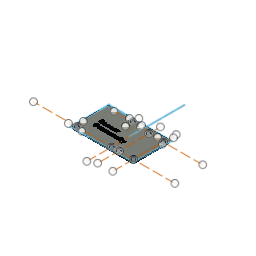
Luftdaten_sensor_holder (Autodesk Fusion 360 design; units mm, degrees)
Autodesk Fusion 360 part; units mm, degrees
sketch "Sketch1" plane through (0, 0, 0) normal (0, 1, 0) x (1, 0, 0)
  circle A0 centre (32.103, -20.4759) radius 1.325
  circle A1 centre (92.103, -20.4759) radius 1.325
  circle A2 centre (73.103, 34.5241) radius 1.325
  line L0 (100.7373, -20.4759) -> (-42.1485, -20.4759) construction
  circle A3 centre (73.103, 34.5241) radius 2.325
  circle A4 centre (92.103, -20.4759) radius 2.325
  circle A5 centre (32.103, -20.4759) radius 2.325
  circle A6 centre (104.103, 31.0241) radius 1.325
  circle A7 centre (129.103, 31.0241) radius 1.325
  circle A8 centre (104.103, -20.4759) radius 1.325
  circle A9 centre (129.103, -20.4759) radius 1.325
  line L1 (104.103, 50.9293) -> (104.103, -56.6428) construction
  line L2 (129.103, -55.7039) -> (129.103, 53.0753) construction
  circle A10 centre (104.103, 31.0241) radius 2.325
  circle A11 centre (104.103, -20.4759) radius 2.325
  circle A12 centre (129.103, -20.4759) radius 2.325
  circle A13 centre (129.103, 31.0241) radius 2.325
  line L3 (196.6906, 31.0241) -> (105, 31.0241) construction
  line L4 (200.3141, -20.4759) -> (105.3141, -20.4759) construction
  line L5 (92.103, -63.1974) -> (92.103, 103.9329) construction
  line L6 (92.103, 103.9329) -> (92.103, 10)
  line L7 (71.8078, 34.4241) -> (41, 34.4241) construction
  line L8 (73.103, 22) -> (73.103, 45) construction
  line L9 (134.428, -25.8009) -> (26.778, -25.8009)
  line L10 (26.778, -25.8009) -> (26.778, 39.8491)
  line L11 (26.778, 39.8491) -> (134.428, 39.8491)
  line L12 (134.428, 39.8491) -> (134.428, -25.8009)
  line L13 (29.778, -7) -> (29.778, -20.4759) construction
  line L14 (20, -22.8009) -> (43, -22.8009) construction
  line L15 (87, 33.3491) -> (117, 33.3491) construction
  line L16 (131.428, 46) -> (131.428, 27) construction
  line L17 (86, 36.8491) -> (65, 36.8491) construction
  dimension "d1" = 2.65
  dimension "d3" = 2.65
  dimension "d4" = 2.65
  dimension "d5" = 60
  dimension "d10" = 41
  dimension "d11" = 55
  dimension "d13" = 1
  dimension "d14" = 1
  dimension "d15" = 1
  dimension "d18" = 2.65
  dimension "d19" = 2.65
  dimension "d20" = 2.65
  dimension "d21" = 2.65
  dimension "d22" = 1
  dimension "d23" = 1
  dimension "d24" = 1
  dimension "d25" = 1
  dimension "d26" = 25
  dimension "d27" = 51.5
  dimension "d28" = 12
  dimension "d31" = 3
  dimension "d32" = 3
  dimension "d34" = 3
  dimension "d42" = 3
  constraint horizontal L0
  constraint coincident A0.centre L0
  constraint coincident A1.centre L0
  constraint vertical L1
  constraint vertical L2
  constraint coincident A7.centre L2
  constraint coincident A9.centre L2
  constraint coincident A8.centre L1
  constraint coincident A6.centre L1
  constraint horizontal L3
  constraint coincident A6.centre L3
  constraint coincident A7.centre L3
  constraint horizontal L4
  constraint coincident A8.centre L4
  constraint coincident A9.centre L4
  constraint perpendicular L0 L5
  constraint coincident L5 L6.end
  constraint coincident A1.centre L5
  constraint horizontal L7
  constraint vertical L8
  constraint coincident A2.centre L8
  constraint horizontal L9
  constraint vertical L10
  constraint horizontal L11
  constraint vertical L12
  constraint coincident L0 L13.end
  constraint perpendicular L0 L13
  constraint tangent A5 L13
  constraint perpendicular L10 L14
  constraint tangent A5 L14
  constraint perpendicular L5 L15
  constraint tangent A10 L15
  constraint perpendicular L11 L16
  constraint tangent A13 L16
  constraint collinear L0 L4
  constraint horizontal L17
  constraint tangent A3 L17
  measures "d1" diameter of A2
  measures "d3" diameter of A0
  measures "d4" diameter of A1
  measures "d5" distance of A0.centre A1.centre
  measures "d10" horizontal distance of A0.centre A2.centre
  measures "d11" vertical distance of A0.centre A2.centre
  measures "d18" diameter of A6
  measures "d19" diameter of A7
  measures "d20" diameter of A8
  measures "d21" diameter of A9
  measures "d26" distance of L1 L2
  measures "d27" distance of L3 L4
  measures "d28" horizontal distance of A1.centre A6.centre
  measures "d31" distance of L10 L13
  measures "d32" distance of L9 L14
  measures "d34" distance of L12 L16
  measures "d42" distance of L11 L17
extrude "Extrude2" add sketch "Sketch1" against normal blind 1.5 contours A0 | A1 | A2 | A3 | A4 | A5 | A6 | A7 | A8 | A9 | A10 | A11 | A12 | A13 | L9 L10 L11 L12
extrude "Extrude1" add sketch "Sketch1" along normal blind 4 contours A3 | A4 | A5 | A10 | A11 | A12 | A13
sketch "Sketch2" plane through (0, 0, 0) normal (0, 1, 0) x (1, 0, 0)
  line L0 (42.778, 4.8491) -> (80.767, 4.8491) construction
  line L1 (80.767, 4.8491) -> (80.767, 14.8491) construction
  line L2 (80.767, 14.8491) -> (42.778, 14.8491) construction
  line L3 (42.778, 14.8491) -> (42.778, 4.8491) construction
  line L4 (42.778, -7.1509) -> (101.4652, -7.1509) construction
  line L5 (101.4652, -7.1509) -> (101.4652, 2.8491) construction
  line L6 (101.4652, 2.8491) -> (42.778, 2.8491) construction
  line L7 (42.778, 2.8491) -> (42.778, -7.1509) construction
  line L8 (26.778, -25.8009) -> (26.778, 39.8491)
  line L9 (26.778, 39.8491) -> (134.428, 39.8491)
  dimension "d36" = 16
  dimension "d37" = 16
  dimension "d38" = 2
  dimension "d39" = 25
  text T0 "Sensor" font "Arial" height 10 bold align ink ink in box 0 x 0 at (42.778, 4.8491) x (1, 0) y (0, 1) spacing 1 height is em
  text T1 "Community" font "Arial" height 10 bold align ink ink in box 0 x 0 at (42.778, -7.1509) x (1, 0) y (0, 1) spacing 1 height is em
  constraint perpendicular L0 L1
  constraint parallel L0 L2
  constraint parallel L1 L3
  constraint perpendicular L4 L5
  constraint parallel L4 L6
  constraint parallel L5 L7
  measures "d36" distance of L3 L8
  measures "d37" distance of L7 L8
  measures "d38" distance of L0 L6
  measures "d39" distance of L2 L9
extrude "Extrude3" add sketch "Sketch2" along normal blind 0.5 text T0 T1
fillet "Fillet1" radius 6 4 edges at (134.428, -0.75, -39.8491) (134.428, -0.75, 25.8009) (26.778, -0.75, 25.8009) (26.778, -0.75, -39.8491)
equation "d1 = screw_size"
equation "screw_size = 2.65 mm"
equation "d3 = screw_size"
equation "d4 = screw_size"
equation "screw_wall_thickness = 1 mm"
equation "d13 = screw_wall_thickness"
equation "d14 = screw_wall_thickness"
equation "d15 = screw_wall_thickness"
equation "d18 = screw_size"
equation "d19 = screw_size"
equation "d20 = screw_size"
equation "d21 = screw_size"
equation "d22 = screw_wall_thickness"
equation "d23 = screw_wall_thickness"
equation "d24 = screw_wall_thickness"
equation "d25 = screw_wall_thickness"
equation "d32 = d31"
equation "d34 = d31"
equation "d37 = d36"
equation "d42 = d31"
